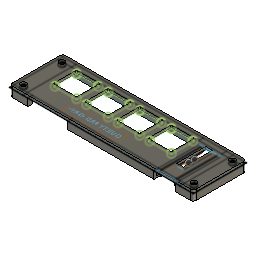
case-top (Autodesk Fusion 360 design; units mm, degrees)
part number: 2025-11-22-15-29-30-254
Autodesk Fusion 360 part; units mm, degrees
sketch "layout" plane through (0, 0, 0) normal (0, 0, 1) x (1, 0, 0)
  line L0 (0.025, -13.525) -> (0.025, -0.525)
  line L1 (14.025, -13.525) -> (14.025, -0.525)
  line L2 (0.525, -14.025) -> (13.525, -14.025)
  line L3 (0.525, -0.025) -> (13.525, -0.025)
  arc A0 (0.025, -13.525) -> (0.525, -14.025) centre (0.525, -13.525) ccw
  arc A1 (0.525, -0.025) -> (0.025, -0.525) centre (0.525, -0.525) ccw
  arc A2 (13.525, -14.025) -> (14.025, -13.525) centre (13.525, -13.525) ccw
  arc A3 (14.025, -0.525) -> (13.525, -0.025) centre (13.525, -0.525) ccw
  line L4 (19.075, -13.525) -> (19.075, -0.525)
  line L5 (33.075, -13.525) -> (33.075, -0.525)
  line L6 (19.575, -14.025) -> (32.575, -14.025)
  line L7 (19.575, -0.025) -> (32.575, -0.025)
  arc A4 (19.075, -13.525) -> (19.575, -14.025) centre (19.575, -13.525) ccw
  arc A5 (19.575, -0.025) -> (19.075, -0.525) centre (19.575, -0.525) ccw
  arc A6 (32.575, -14.025) -> (33.075, -13.525) centre (32.575, -13.525) ccw
  arc A7 (33.075, -0.525) -> (32.575, -0.025) centre (32.575, -0.525) ccw
  line L8 (38.125, -13.525) -> (38.125, -0.525)
  line L9 (52.125, -13.525) -> (52.125, -0.525)
  line L10 (38.625, -14.025) -> (51.625, -14.025)
  line L11 (38.625, -0.025) -> (51.625, -0.025)
  arc A8 (38.125, -13.525) -> (38.625, -14.025) centre (38.625, -13.525) ccw
  arc A9 (38.625, -0.025) -> (38.125, -0.525) centre (38.625, -0.525) ccw
  arc A10 (51.625, -14.025) -> (52.125, -13.525) centre (51.625, -13.525) ccw
  arc A11 (52.125, -0.525) -> (51.625, -0.025) centre (51.625, -0.525) ccw
  line L12 (57.175, -13.525) -> (57.175, -0.525)
  line L13 (71.175, -13.525) -> (71.175, -0.525)
  line L14 (57.675, -14.025) -> (70.675, -14.025)
  line L15 (57.675, -0.025) -> (70.675, -0.025)
  arc A12 (57.175, -13.525) -> (57.675, -14.025) centre (57.675, -13.525) ccw
  arc A13 (57.675, -0.025) -> (57.175, -0.525) centre (57.675, -0.525) ccw
  arc A14 (70.675, -14.025) -> (71.175, -13.525) centre (70.675, -13.525) ccw
  arc A15 (71.175, -0.525) -> (70.675, -0.025) centre (70.675, -0.525) ccw
  line L16 (-12.6365, 4.226) -> (98.1475, 4.226)
  line L17 (98.1475, 4.226) -> (98.1475, -27.774)
  line L18 (98.1475, -27.774) -> (-12.6365, -27.774)
  line L19 (-12.6365, -27.774) -> (-12.6365, 4.226)
  line L20 (85.8249, -0.274) -> (75.9249, -0.274)
  line L21 (75.9249, -0.274) -> (75.9249, -26.274)
  line L22 (75.9249, -26.274) -> (85.8249, -26.274)
  line L23 (85.8249, -26.274) -> (85.8249, -0.274)
  line L24 (85.8249, -0.274) -> (75.9249, -26.274) construction
  line L25 (75.9249, -0.274) -> (85.8249, -26.274) construction
  line L26 (76.5749, -26.274) -> (76.5749, -0.274)
  line L27 (85.1749, -26.274) -> (85.1749, -0.274)
  line L28 (82.875, -18.454) -> (78.875, -18.454)
  line L29 (78.875, -18.454) -> (78.875, -0.954)
  line L30 (78.875, -0.954) -> (82.875, -0.954)
  line L31 (82.875, -0.954) -> (82.875, -18.454)
  line L32 (82.875, -18.454) -> (78.875, -0.954) construction
  line L33 (78.875, -18.454) -> (82.875, -0.954) construction
  line L34 (-12.6365, 1.526) -> (98.1475, 1.526)
  line L35 (86.1475, 1.526) -> (86.1475, 4.226)
  line L36 (72.1475, 1.526) -> (72.1475, 4.226)
  circle A16 centre (94.1475, -23.374) radius 1.7
  circle A17 centre (94.1475, -0.174) radius 1.7
  circle A18 centre (-8.6365, -23.374) radius 1.7
  circle A19 centre (-8.6365, -0.174) radius 1.7
  line L37 (90.1475, -27.774) -> (90.1475, 4.226)
  line L38 (-4.6365, -27.774) -> (-4.6365, 4.226)
  line L39 (98.1475, -25.074) -> (-12.6365, -25.074)
  line L40 (74.4249, -25.074) -> (74.4249, -27.774)
  line L41 (87.3249, -27.774) -> (87.3249, -25.074)
  line L42 (-1.6365, -27.774) -> (-1.6365, -25.074)
  line L43 (22.3635, -27.774) -> (22.3635, -25.074)
  line L44 (75.9249, -26.274) -> (74.4249, -26.274)
  line L45 (74.4249, -26.274) -> (74.4249, -0.274)
  line L46 (74.4249, -0.274) -> (75.9249, -0.274)
  line L47 (75.9249, -0.274) -> (75.9249, -26.274)
  line L48 (85.8249, -26.274) -> (87.3249, -26.274)
  line L49 (87.3249, -26.274) -> (87.3249, -0.2454)
  line L50 (87.3249, -0.2454) -> (85.8249, -0.2454)
  line L51 (85.8249, -0.2454) -> (85.8249, -26.274)
  point P0 (80.8749, -13.274)
  point P1 (80.875, -9.704)
  dimension "d1" = 110.784
  dimension "d2" = 32
  dimension "d3" = 12.6615
  dimension "d4" = 13.749
  dimension "d10" = 9.9
  dimension "d11" = 26
  dimension "d14" = 0.65
  dimension "d15" = 0.65
  dimension "d16" = 0.0001
  dimension "d17" = 4
  dimension "d18" = 9.43
  dimension "d19" = 17.5
  dimension "d20" = 9.7
  dimension "d22" = 2.7
  dimension "d23" = 12
  dimension "d24" = 14
  dimension "d25" = 3.4
  dimension "d26" = 4.4
  dimension "d27" = 4
  dimension "d28" = 3.4
  dimension "d29" = 4
  dimension "d30" = 4.4
  dimension "d31" = 3.4
  dimension "d32" = 4.4
  dimension "d33" = 4
  dimension "d34" = 3.4
  dimension "d35" = 4.4
  dimension "d36" = 4
  dimension "d37" = 8
  dimension "d38" = 8
  dimension "d39" = 2.7
  dimension "d40" = 1.5
  dimension "d41" = 1.5
  dimension "d42" = 11
  dimension "d43" = 24
  dimension "d48" = 1.5
  dimension "d49" = 1.5
  constraint horizontal L16
  constraint vertical L17
  constraint horizontal L18
  constraint vertical L19
  constraint horizontal L20
  constraint perpendicular L20 L21
  constraint parallel L20 L22
  constraint parallel L21 L23
  constraint coincident L24 P0
  constraint coincident L25 P0
  constraint coincident L22 L26.start
  constraint coincident L20 L26.end
  constraint perpendicular L20 L26
  constraint coincident L22 L27.start
  constraint coincident L20 L27.end
  constraint perpendicular L20 L27
  constraint horizontal L28
  constraint perpendicular L28 L29
  constraint parallel L28 L30
  constraint parallel L29 L31
  constraint coincident L32 P1
  constraint coincident L33 P1
  constraint coincident L19 L34.start
  constraint coincident L17 L34.end
  constraint perpendicular L17 L34
  constraint coincident L34 L35.start
  constraint coincident L16 L35.end
  constraint perpendicular L16 L35
  constraint coincident L34 L36.start
  constraint coincident L16 L36.end
  constraint perpendicular L16 L36
  constraint coincident L18 L37.start
  constraint coincident L16 L37.end
  constraint perpendicular L16 L37
  constraint coincident L18 L38.start
  constraint coincident L16 L38.end
  constraint perpendicular L16 L38
  constraint coincident L17 L39.start
  constraint coincident L19 L39.end
  constraint perpendicular L19 L39
  constraint coincident L39 L40.start
  constraint coincident L18 L40.end
  constraint perpendicular L18 L40
  constraint coincident L18 L41.start
  constraint coincident L39 L41.end
  constraint perpendicular L39 L41
  constraint coincident L18 L42.start
  constraint coincident L39 L42.end
  constraint perpendicular L39 L42
  constraint coincident L18 L43.start
  constraint coincident L39 L43.end
  constraint perpendicular L39 L43
  constraint horizontal L44
  constraint vertical L45
  constraint horizontal L46
  constraint vertical L47
  constraint horizontal L48
  constraint vertical L49
  constraint horizontal L50
  constraint vertical L51
  measures "d1" distance of L16.start L16.end
  measures "d2" distance of L16 L18
  measures "d3" distance of L0 L19
  measures "d4" distance of L2 L18
  measures "d10" distance of L21 L23
  measures "d11" distance of L20 L22
  measures "d14" distance of L21 L26
  measures "d15" distance of L23 L27
  measures "d16" horizontal distance of P0 P1
  measures "d17" distance of L29 L31
  measures "d18" distance of L20 P1
  measures "d19" distance of L28 L30
  measures "d20" distance of L13 P1
  measures "d22" distance of L16 L34
  measures "d23" distance of L17 L35
  measures "d24" distance of L35 L36
  measures "d25" diameter of A16
  measures "d26" distance of L18 A16.centre
  measures "d27" distance of L17 A16.centre
  measures "d28" diameter of A17
  measures "d29" distance of L17 A17.centre
  measures "d30" distance of L16 A17.centre
  measures "d31" diameter of A18
  measures "d32" distance of L18 A18.centre
  measures "d33" distance of L19 A18.centre
  measures "d34" diameter of A19
  measures "d35" distance of L16 A19.centre
  measures "d36" distance of L19 A19.centre
  measures "d37" distance of L17 L37
  measures "d38" distance of L19 L38
  measures "d39" distance of L18 L39
  measures "d40" distance of L23 L41
  measures "d41" distance of L21 L40
  measures "d42" distance of L19 L42
  measures "d43" distance of L42 L43
  measures "d48" distance of L45 L47
  measures "d49" distance of L22.end L48.end
extrude "Extrude1" add sketch "layout" along normal blind 1.5 makes body 1
extrude "Extrude2" add sketch "layout" against normal blind 4.5 separate body contours L16 L19 L34 L38 | L16 L34 L36 L38 | L19 L34 L38 L39 | L18 L19 L38 L39 | L16 L34 L35 L37 | L18 L38 L39 L42 | L16 L17 L34 L37 | L17 L34 L37 L39 | L18 L39 L40 L43 L45 | L17 L18 L37 L39 | L18 L37 L39 L41 L49 makes body 2 at (18.2915, 3.326, 0) makes body 3 at (92.6881, 3.3118, 0) makes body 4 at (57.0711, -25.074, -1.5)
extrude "Extrude3" add sketch "layout" against normal blind 2 separate body contours L21 L39 L45 L46 L47 | L21 L39 L40 L44 L45 L47 | L23 L39 L41 L48 L49 L51 | L23 L39 L49 L50 L51 makes body 5 at (87.3249, -17.5978, -1.3333) makes body 6 at (74.4249, -17.6073, -0.6667)
sketch "daughterboard carrier overhang" plane through (0, 0, -2) normal (0, 0, -1) x (1, 0, 0)
  line L0 (74.4249, 0.274) -> (75.9249, 0.274)
  line L1 (75.9249, 0.274) -> (75.9249, 26.274)
  line L2 (75.9249, 26.274) -> (74.4249, 26.274)
  line L3 (74.4249, 26.274) -> (74.4249, 0.274)
  line L4 (75.9249, 0.274) -> (76.5749, 0.274)
  line L5 (76.5749, 0.274) -> (76.5749, 26.274)
  line L6 (76.5749, 26.274) -> (75.9249, 26.274)
  line L7 (75.9249, 26.274) -> (75.9249, 0.274)
  line L8 (75.9249, 26.274) -> (74.4249, 26.274)
  line L9 (74.4249, 26.274) -> (74.4249, 0.274)
  line L10 (74.4249, 0.274) -> (75.9249, 0.274)
  line L11 (75.9249, 0.274) -> (75.9249, 26.274)
  line L12 (85.1749, 0.274) -> (85.8249, 0.274)
  line L13 (85.8249, 0.274) -> (85.8249, 26.274)
  line L14 (85.8249, 26.274) -> (85.1749, 26.274)
  line L15 (85.1749, 26.274) -> (85.1749, 0.274)
  line L16 (85.8249, 0.274) -> (87.3249, 0.274)
  line L17 (87.3249, 0.274) -> (87.3249, 26.274)
  line L18 (87.3249, 26.274) -> (85.8249, 26.274)
  line L19 (85.8249, 26.274) -> (85.8249, 0.274)
  dimension "d52" = 0.65
  dimension "d60" = 0.65
  dimension "d61" = 26
  dimension "d62" = 8.6
  dimension "d63" = 1.5
  dimension "d64" = 26
  constraint horizontal L4
  constraint vertical L5
  constraint horizontal L6
  constraint vertical L7
  constraint coincident L0.end L1.start
  constraint horizontal L8
  constraint vertical L9
  constraint horizontal L10
  constraint vertical L11
  constraint coincident L0.start L3.end
  constraint coincident L1.end L2.start
  constraint horizontal L12
  constraint vertical L13
  constraint horizontal L14
  constraint vertical L15
  constraint horizontal L16
  constraint vertical L17
  constraint horizontal L18
  constraint vertical L19
  measures "d52" distance of L5 L7
  measures "d60" distance of L12.start L12.end
  measures "d61" distance of L12.start L14.end
  measures "d62" distance of L5 L15
  measures "d63" distance of L12.end L16.end
  measures "d64" distance of L12.end L13.end
extrude "Extrude4" add sketch "daughterboard carrier overhang" along normal blind 1 bodies 3 4 5 6
fillet "Fillet1" radius 1.7 8 edges at (98.1475, -27.774, 0.75) (98.1475, 4.226, 0.75) (-12.6365, 4.226, 0.75) (-12.6365, -27.774, 0.75) (-12.6365, 4.226, -2.25) (-12.6365, -27.774, -2.25) (98.1475, -27.774, -2.25) (98.1475, 4.226, -2.25) on bodies 1 2 3
sketch "Sketch3" plane through (0, 0, 0) normal (0, 0, 1) x (1, 0, 0)
  line L0 (48, -24) -> (15, -24) construction
  line L1 (15, -24) -> (15, -17) construction
  line L2 (15, -17) -> (48, -17) construction
  line L3 (48, -17) -> (48, -24) construction
  dimension "d69" = 2.5
  text T0 "GUILTY PAD -GAY-" font "Arial" height 2.5 align centre middle in box 33 x 7 at (48, -24) x (-1, 0) y (0, 1) spacing 1 kerned
extrude "Extrude6" cut sketch "Sketch3" along normal blind 0.2 text T0 bodies 1
equation "d70 = 'GUILTY PAD -GAY-'"
